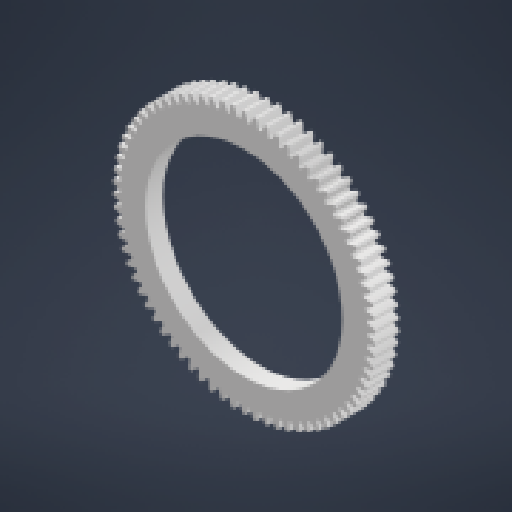
# Autodesk Inventor part: Ring Gear Base
Saved by Autodesk Inventor 2023 (Build 270158000, 158)
## iProperties
Created: 2023-08-11
Part Number: Ring Gear Base
Material: Generic
Document SubType Name: Modeling
Designer: Izack Waczko
Density: 1 g/cm^3
Appearance: Default
Author: Izack Waczko
Autodesk Inventor part; units mm, degrees
ref_plane "YZ Plane" through (0, 0, 0) normal (1, 0, 0) x (0, 1, 0)
ref_plane "XZ Plane" through (0, 0, 0) normal (0, 1, 0) x (-1, 0, 0)
ref_plane "XY Plane" through (0, 0, 0) normal (0, 0, 1) x (1, 0, 0)
sketch "Sketch1" plane through (0, 0, 0) normal (0, 0, 1) x (1, 0, 0)
  line L0 (-44.3976, 4.5) -> (-44.3976, -4.5) construction
  line L1 (3.4024, -4.5) -> (3.4024, 4.5) construction
  line L2 (3.4024, 0) -> (-44.3976, 0) construction
  circle A0 centre (-20.4976, 0) radius 28.5
  circle A1 centre (-20.4976, 0) radius 38.5
  point P0 (0, 0)
  dimension "d0" = 57
  dimension "d1" = 10
  constraints: 3 midpoint, 2 centre point, 2 end point
  measures "d0" diameter of A0
  measures "d1" radial gap between concentric circles of A0 A1
extrude "Extrusion1" add sketch "Sketch1" along normal blind 7
sketch "Sketch2" plane through (-20.4976, 0, 0) normal (0, 0, -1) x (-1, 0, 0)
  circle A0 centre (0, 0) radius 35.5
  circle A1 centre (0, 0) radius 28.5 projected
  point P0 (-20.4976, 0)
  dimension "d4" = 71
  constraints: 1 centre point
  measures "d4" diameter of A0
extrude "Extrusion2" cut sketch "Sketch2" against normal blind 1.9 contours A0 | A1
spur gear teeth "Spur Gear1" teeth 74 pitch diameter 74 tip diameter 76 root diameter 71.5 face width 8 trims to tip circle yes start plane through (-20.4976, 0, 7) normal (0, 0, 1) x (1, 0, 0)
sketch "Sketch3" plane through (0, 0, 7) normal (0, 0, 1) x (1, 0, 0)
  circle A0 centre (-20.4976, 0) radius 28.5 projected
  line L0 (3.7356, -15) -> (-44.7309, -15) construction
  circle A1 centre (-40.1842, -15) radius 3.75
  circle A2 centre (-40.1842, -15) radius 1.6
  circle A3 centre (-20.4976, 0) radius 28.5 construction
  line L1 (8.0024, 0) -> (-48.9976, 0) construction
  line L2 (-43.167, -17.2727) -> (-38.6451, -23.2075)
  line L3 (-38.6451, -23.2075) -> (-38.6451, -18.4196)
  line L4 (-43.167, -17.2727) -> (-36.7444, -12.3791) construction
  line L5 (-47.689, -11.338) -> (-43.0728, -12.6086)
  line L6 (-47.689, -11.338) -> (-43.167, -17.2727)
  point P0 (0, 0)
  point P1 (-46.5011, -11.6649)
  point P2 (-43.167, -17.2727)
  point P3 (-38.6451, -21.9754)
  dimension "d7" = 15
  dimension "d9" = 7.5
  dimension "d10" = 3.2
  constraints: 14 end point, 7 point on circle, 4 tangent, 2 centre point, 2 horizontal, 2 symmetric about line, 1 coincident, 1 point on line, 1 vertical
  measures "d7" distance from line of L0 A0.centre
  measures "d9" diameter of A1
  measures "d10" diameter of A2
extrude "Extrusion3" add sketch "Sketch3" against normal blind 3 contours L5 A1 A0 | A0 A1 L3 | A1
fillet "Fillet1" radius 2 4 edges at (-38.6451, -18.4196, 5.5) (-43.0728, -12.6086, 5.5) (-46.5011, -11.6649, 5.5) (-38.6451, -21.9754, 5.5)
pattern_circular "Circular Pattern1" count 4 over 360 about axis through (-20.4976, 0, 0) along (0, 0, 1) of "Extrusion3"
body "Solid1"
